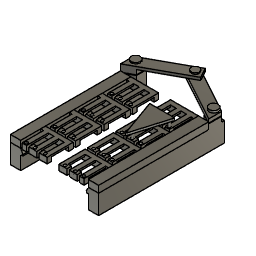
GuitarBuddy (Autodesk Fusion 360 design; units mm, degrees)
Autodesk Fusion 360 part; units mm, degrees
note: some values were not read from the file. Chosen so that the rebuilt part matches the saved one: a direction; which face or edge a step refers to. Set by a fixed rule: which sketch regions a step uses.
sketch "Sketch1" plane through (0, 0, 0) normal (0, 0, 1) x (1, 0, 0)
  line L0 (0, 0) -> (4.5, 0)
  line L1 (4.5, 0) -> (4.5, 101.6)
  line L2 (4.5, 101.6) -> (0, 101.6)
  line L3 (0, 101.6) -> (0, 0)
  line L4 (4.5, 101.6) -> (41, 101.6) construction
  line L5 (41, 101.6) -> (41, 121.6) construction
  line L6 (41, 121.6) -> (4.5, 101.6)
  line L7 (41, 121.6) -> (36.1947, 130.3698)
  line L8 (36.1947, 130.3698) -> (0, 110.5371)
  line L9 (0, 110.5371) -> (0, 101.6)
  line L10 (4.5, 101.6) -> (4.5, 110.5371)
  line L11 (4.5, 110.5371) -> (0, 110.5371)
  line L12 (-4.5, 110.5371) -> (0, 110.5371)
  line L13 (-4.5, 101.6) -> (-4.5, 110.5371)
  line L14 (-4.5, 0) -> (-4.5, 101.6)
  line L15 (0, 0) -> (-4.5, 0)
  line L16 (0, 110.5371) -> (-4.5, 108.0713)
  line L17 (4.5, 101.6) -> (-4.5, 96.6685)
  line L18 (4.5, 101.6) -> (-4.5, 101.6)
  line L19 (34.2124, 123.5822) -> (34.2124, 117.8808) construction
  line L20 (63.9249, 101.6) -> (72.9249, 96.6685)
  line L21 (63.9249, 101.6) -> (72.9249, 101.6) construction
  line L22 (27.4249, 121.6) -> (32.2302, 130.3698)
  line L23 (68.4249, 110.5371) -> (68.4249, 101.6)
  line L24 (63.9249, 110.5371) -> (68.4249, 110.5371)
  line L25 (68.4249, 110.5371) -> (72.9249, 108.0713)
  line L26 (72.9249, 0) -> (72.9249, 101.6)
  line L27 (72.9249, 101.6) -> (72.9249, 110.5371)
  line L28 (63.9249, 101.6) -> (27.4249, 101.6) construction
  line L29 (63.9249, 0) -> (63.9249, 101.6)
  line L30 (68.4249, 101.6) -> (68.4249, 0)
  line L31 (27.4249, 121.6) -> (63.9249, 101.6)
  line L32 (34.2124, 123.5822) -> (34.2124, 117.8808) construction
  line L33 (32.2302, 130.3698) -> (68.4249, 110.5371)
  line L34 (63.9249, 101.6) -> (68.4249, 101.6) construction
  line L35 (72.9249, 110.5371) -> (68.4249, 110.5371)
  line L36 (27.4249, 101.6) -> (27.4249, 121.6) construction
  line L37 (63.9249, 101.6) -> (63.9249, 110.5371)
  line L38 (68.4249, 0) -> (72.9249, 0)
  line L39 (68.4249, 0) -> (63.9249, 0)
  circle A0 centre (34.2124, 123.5822) radius 2.7
  circle A1 centre (34.2124, 123.5822) radius 3
  circle A2 centre (34.2124, 123.5822) radius 3.45
  line L40 (-4.5, 105.5371) -> (4.5, 105.5371) construction
  circle A3 centre (0, 105.5371) radius 3
  circle A4 centre (0, 105.5371) radius 4
  circle A5 centre (0, 105.5371) radius 2.4
  line L41 (72.9249, 105.5371) -> (63.9249, 105.5371) construction
  circle A6 centre (68.4249, 105.5371) radius 2.4
  circle A7 centre (68.4249, 105.5371) radius 3
  circle A8 centre (68.4249, 105.5371) radius 4
  point P0 (68.4249, 0)
  dimension "d3" = 4.5
  dimension "d4" = 101.6
  dimension "d9" = 36.5
  dimension "d11" = 20
  dimension "d13" = 10
  dimension "d19" = 5
  dimension "d20" = 5
  dimension "d300" = 6
  dimension "d301" = 6.9
  dimension "d302" = 5.4
  dimension "d337" = 5
  dimension "d338" = 6
  dimension "d339" = 8
  dimension "d340" = 4.8
  constraint horizontal L0
  constraint vertical L1
  constraint horizontal L2
  constraint vertical L3
  constraint coincident L0.start L3.end
  constraint perpendicular L1 L4
  constraint perpendicular L4 L5
  constraint perpendicular L6 L7
  constraint perpendicular L2 L9
  constraint parallel L6 L8
  constraint perpendicular L4 L10
  constraint perpendicular L9 L11
  constraint symmetric L0.start L9 L3.end
  constraint symmetric L0.end L9 L14.start
  constraint symmetric L1.end L9 L13.start
  constraint symmetric L8.end L9 L11.end
  constraint symmetric L9 L10.end L12.start
  constraint coincident L9 L8.end
  constraint coincident L13 L16.end
  constraint collinear L8 L16
  constraint coincident L14 L17.end
  constraint collinear L6 L17
  constraint coincident L6 L19.end
  constraint vertical L19
  constraint symmetric L0.start L19 L30.end
  constraint symmetric L0.start L19 P0
  constraint symmetric L0.end L19 L29.start
  constraint symmetric L1.end L19 L20.start
  constraint symmetric L2.end L19 L23.end
  constraint symmetric L4.end L19 L28.end
  constraint symmetric L5.end L19 L22.start
  constraint symmetric L7.end L19 L22.end
  constraint symmetric L8.end L19 L23.start
  constraint symmetric L10.end L19 L24.start
  constraint symmetric L12.start L19 L27.end
  constraint symmetric L13.start L19 L21.end
  constraint symmetric L14.start L19 L26.start
  constraint symmetric L16.end L19 L25.end
  constraint symmetric L17.end L19 L20.end
  constraint symmetric L32.start L19 A0.centre
  constraint symmetric L32.end L19 L19.end
  constraint concentric A1 A2
  constraint concentric A0 A2
  constraint coincident L19.start L32.start
  constraint coincident L13 L40.start
  constraint coincident L10 L40.end
  constraint horizontal L40
  constraint midpoint L40 A3.centre
  constraint concentric A3 A4
  constraint concentric A3 A5
  constraint symmetric L19 L40.start L41.start
  constraint symmetric L19 L40.end L41.end
  constraint symmetric L19 A3 A7
  constraint symmetric L19 A4 A8
  constraint symmetric L19 A5 A6
  measures "d3" distance of L0.start L0.end
  measures "d4" distance of L0.start L2.end
  measures "d9" distance of L1.end L4.end
  measures "d11" distance of L4.end L5.end
  measures "d13" distance of L5.end L7.end
  measures "d19" distance of L8 L19.start
  measures "d20" distance of L7 L19.start
  measures "d300" diameter of A1
  measures "d301" diameter of A2
  measures "d302" diameter of A0
  measures "d337" distance of L12 L40
  measures "d338" diameter of A3
  measures "d339" diameter of A4
  measures "d340" diameter of A5
extrude "Extrude2" add sketch "Sketch1" along normal blind 3.175 from surface at 5 contours L3 L14 L17 L18 A4 | L2 L3 L17 L18 A4 | L6 L8 L10 L11 L22 L31 | L2 L9 L10 L11 L18 A4 | L3 L18 A4 | L2 L3 L18 A4 | L2 L9 L18 A3 A4 | L6 L7 L8 L22 L31 L33 | L9 L18 A3 A4 | L9 L13 L16 L18 A4 | L9 A3 A5 | L9 A3 A5 | L7 L8 L33 | L9 A5 | L9 A5 | A2 makes body 1 in component "LeftHandleBar"
extrude "Extrude4" add sketch "Sketch1" along normal mid plane 6.35 from surface at 8.175 separate body contours A0 makes body 2 in component "CenterRivot"
extrude "Extrude5" add sketch "Sketch1" along normal blind 1.5875 from surface at 11.35 separate body contours A0 | A1 | A2 makes body 3 in component "CenterRivot"
extrude "Extrude6" add sketch "Sketch1" against normal blind 1.5875 from surface at 5 separate body contours A0 | A1 | A2 makes body 4 in component "CenterRivot"
extrude "Extrude1" add sketch "Sketch1" against normal blind 17 separate body contours L0 L1 L3 L17 | L2 L3 L17 L18 A4 | L2 L9 L10 L11 L18 A4 | L2 L3 L18 A4 | L2 L9 L18 A3 A4 | L9 A3 A5 | L9 A5 picked at (1.628, 103.2671) picked at (0.5577, 104.777) makes body 5
copy_body "Body->Comp1" bodies 5 removing the originals makes body 6 in component "LeftHandle"
sketch "Sketch2" plane through (4.5, 0, 0) normal (1, 0, 0) x (0, 1, 0)
  line L0 (109.1262, 0) -> (0, 0)
  line L1 (0, 0) -> (0, -19.05)
  line L2 (0, -19.05) -> (109.1262, -19.05)
  line L3 (109.1262, -19.05) -> (109.1262, 0)
  line L4 (0, 0) -> (3.81, 0)
  line L5 (3.81, 0) -> (3.81, -5)
  line L6 (3.81, -5) -> (0, -5)
  line L7 (0, -5) -> (0, 0)
  line L8 (101.6, 0) -> (97.79, 0)
  line L9 (97.79, 0) -> (97.79, -5)
  line L10 (97.79, -5) -> (101.6, -5)
  line L11 (101.6, -5) -> (101.6, 0)
  line L12 (110.5371, 0) -> (0, 0)
  line L13 (0, 0) -> (0, -17)
  line L14 (0, -17) -> (110.5371, -17)
  line L15 (110.5371, -17) -> (110.5371, 0)
  point P0 (101.6, 0)
  dimension "d55" = 3.81
  dimension "d56" = 5
  dimension "d66" = 3.81
  dimension "d67" = 5
  constraint horizontal L4
  constraint vertical L5
  constraint horizontal L6
  constraint vertical L7
  constraint coincident L0.end L1.start
  constraint horizontal L8
  constraint vertical L9
  constraint horizontal L10
  constraint vertical L11
  constraint coincident P0 L8.start
  measures "d55" distance of L0.end L4.end
  measures "d56" distance of L0.end L6.end
  measures "d66" distance of P0 L8.end
  measures "d67" distance of P0 L10.end
extrude "Extrude1'" add sketch "Sketch2" along normal blind 1.905 contours L0 L1 L4 L5 L6 L7 L12 L13 bodies 6 in component "LeftHandle"
extrude "Extrude14" add sketch "Sketch2" along normal blind 2.905 contours L0 L8 L9 L10 L11 L12 bodies 6 in component "LeftHandle"
extrude "Extrude3" add 1 faces at (0, 73.6914, -5.6667) along direction (-1, 0, 0) blind 4.5 separate body on bodies 6 makes body 7 in component "LeftHandle"
chamfer "Chamfer1" distance 3.81 distance2 2.905 1 edges at (7.405, 99.695, 0) measured on face at (7.405, 99.06, -1.6667) on bodies 6 in component "LeftHandle"
chamfer "Chamfer2" distance 3.81 distance2 1.905 1 edges at (6.405, 1.905, 0) measured on face at (6.405, 1.27, -3.3333) on bodies 6 in component "LeftHandle"
ref_plane "WorkPlane1" through (0, 0, -1) normal (0, 0, 1) x (1, 0, 0) in component "LeftHandle"
ref_plane "WorkPlane2" through (0, 0, -4) normal (0, 0, 1) x (1, 0, 0) in component "LeftHandle"
sketch "Sketch6" plane through (0, 0, 0) normal (0, 0, 1) x (1, 0, 0)
  line L0 (4.5, 110.5371) -> (0, 110.5371)
  line L1 (0, 110.5371) -> (0, 0)
  line L2 (0, 0) -> (4.5, 0)
  line L3 (4.5, 3.81) -> (4.5, 97.79)
  line L4 (0, 0) -> (0, 110.5371) construction
  line L5 (0, 110.5371) -> (-4.5, 110.5371)
  line L6 (-4.5, 0) -> (0, 0)
  line L7 (41, 121.6) -> (36.1947, 130.3698)
  line L8 (36.1947, 130.3698) -> (-4.5, 108.0713)
  line L9 (-4.5, 108.0713) -> (-4.5, 96.6685)
  line L10 (-4.5, 96.6685) -> (41, 121.6)
  line L11 (34.2124, 123.5822) -> (34.2124, 96.6685) construction
  line L12 (34.2124, 96.6685) -> (4.5, 96.6685) construction
  line L13 (34.2124, 123.5822) -> (36.2124, 123.5822) construction
  line L14 (36.2124, 123.5822) -> (36.2124, 96.6685) construction
  line L15 (36.2124, 96.6685) -> (34.2124, 96.6685) construction
  line L16 (34.2124, 96.6685) -> (34.2124, 123.5822) construction
  line L17 (34.2124, 123.5822) -> (32.2124, 123.5822) construction
  line L18 (32.2124, 123.5822) -> (32.2124, 96.6685) construction
  line L19 (32.2124, 96.6685) -> (34.2124, 96.6685) construction
  line L20 (34.2124, 96.6685) -> (34.2124, 123.5822) construction
  line L21 (32.2124, 96.6685) -> (36.2124, 96.6685) construction
  line L22 (36.2124, 96.6685) -> (36.2124, 0) construction
  line L23 (36.2124, 0) -> (32.2124, 0) construction
  line L24 (32.2124, 0) -> (32.2124, 96.6685) construction
  line L25 (4.5, 96.6685) -> (32.2124, 96.6685) construction
  line L26 (34.2124, 96.6685) -> (34.2124, 0) construction
  circle A0 centre (34.2124, 123.5822) radius 3
  line L27 (34.2124, 123.5822) -> (34.2124, 117.8808)
  line L28 (4.5, 96.6685) -> (32.2124, 96.6685)
  line L29 (32.2124, 96.6685) -> (32.2124, 92.6685)
  line L30 (32.2124, 92.6685) -> (4.5, 92.6685)
  line L31 (4.5, 92.6685) -> (4.5, 96.6685)
  line L32 (11, 92.6685) -> (7, 92.6685)
  line L33 (7, 92.6685) -> (7, 73.6685)
  line L34 (11, 73.6685) -> (11, 92.6685)
  line L35 (11, 73.6685) -> (7, 73.6685)
  circle A1 centre (9, 75.6685) radius 1.25
  line L36 (-4.5, 96.6685) -> (4.5, 96.6685)
  line L37 (7, 77.6685) -> (11, 77.6685)
  line L38 (9, 77.6685) -> (9, 75.6685) construction
  line L39 (11, 77.6685) -> (11, 73.6685) construction
  line L40 (11, 75.6685) -> (9, 75.6685) construction
  line L41 (20, 73.6685) -> (16, 73.6685)
  line L42 (20, 73.6685) -> (20, 92.6685)
  line L43 (16, 77.6685) -> (20, 77.6685)
  line L44 (16, 92.6685) -> (16, 73.6685)
  circle A2 centre (16.5, 75.6685) radius 1.25
  line L45 (20, 75.6685) -> (16.5, 75.6685) construction
  line L46 (20, 92.6685) -> (16, 92.6685)
  line L47 (20, 77.6685) -> (20, 73.6685) construction
  line L48 (16.5, 77.6685) -> (16.5, 75.6685) construction
  line L49 (29, 73.6685) -> (25, 73.6685)
  line L50 (29, 73.6685) -> (29, 92.6685)
  line L51 (25, 77.6685) -> (29, 77.6685)
  line L52 (25, 92.6685) -> (25, 73.6685)
  circle A3 centre (25.5, 75.6685) radius 1.25
  line L53 (29, 75.6685) -> (25.5, 75.6685) construction
  line L54 (29, 92.6685) -> (25, 92.6685)
  line L55 (29, 77.6685) -> (29, 73.6685) construction
  line L56 (25.5, 77.6685) -> (25.5, 75.6685) construction
  line L57 (-4.5, 96.6685) -> (0, 96.6685)
  line L58 (0, 96.6685) -> (0, 0)
  line L59 (0, 0) -> (-4.5, 0)
  line L60 (-4.5, 0) -> (-4.5, 96.6685)
  line L61 (16, 77.6685) -> (13, 77.6685)
  line L62 (13, 77.6685) -> (13, 73.6685)
  line L63 (13, 73.6685) -> (16, 73.6685)
  line L64 (22, 77.6685) -> (22, 73.6685)
  line L65 (22, 73.6685) -> (25, 73.6685)
  line L66 (25, 77.6685) -> (22, 77.6685)
  line L67 (29, 92.6685) -> (29, 96.6685)
  line L68 (13, 77.6685) -> (20, 77.6685) construction
  line L69 (29, 77.6685) -> (22, 77.6685) construction
  line L70 (4.5, 0) -> (4.5, 3.81)
  line L71 (4.5, 97.79) -> (4.5, 101.6)
  line L72 (4.5, 101.6) -> (4.5, 110.5371)
  dimension "d317" = 2
  dimension "d318" = 2
  dimension "d350" = 4
  dimension "d363" = 4
  dimension "d401" = 2.5
  dimension "d436" = 4
  dimension "d437" = 4
  dimension "d438" = 2.5
  dimension "d439" = 4
  dimension "d440" = 4
  dimension "d441" = 2.5
  dimension "d442" = 4
  dimension "d443" = 5
  dimension "d444" = 5
  dimension "d445" = 2.5
  dimension "d446" = 15
  dimension "d447" = 15
  dimension "d449" = 15
  dimension "d465" = 3
  dimension "d466" = 3
  constraint coincident L3 L12.end
  constraint perpendicular L3 L12
  constraint horizontal L13
  constraint vertical L14
  constraint horizontal L15
  constraint vertical L16
  constraint horizontal L17
  constraint vertical L18
  constraint horizontal L19
  constraint vertical L20
  constraint coincident L12 L18.end
  constraint horizontal L21
  constraint vertical L22
  constraint horizontal L23
  constraint vertical L24
  constraint coincident L14.end L15.start
  constraint midpoint L23 L26.end
  constraint horizontal L28
  constraint vertical L29
  constraint vertical L31
  constraint horizontal L32
  constraint vertical L33
  constraint vertical L34
  constraint horizontal L35
  constraint coincident L9.end L10.start
  constraint horizontal L36
  constraint collinear L24 L29
  constraint coincident L33 L37.start
  constraint coincident L34 L37.end
  constraint perpendicular L34 L37
  constraint midpoint L37 L38.start
  constraint coincident A1.centre L38.end
  constraint perpendicular L37 L38
  constraint midpoint L39 L40.start
  constraint perpendicular L39 L40
  constraint horizontal L46
  constraint vertical L44
  constraint vertical L42
  constraint horizontal L41
  constraint coincident L43.start L44
  constraint coincident L43.end L42
  constraint perpendicular L42 L43
  constraint coincident A2.centre L45.end
  constraint perpendicular L43 L48
  constraint midpoint L45.start L47
  constraint perpendicular L45 L47
  constraint horizontal L54
  constraint vertical L52
  constraint vertical L50
  constraint horizontal L49
  constraint coincident L51.start L52
  constraint coincident L51.end L50
  constraint perpendicular L50 L51
  constraint coincident A3.centre L53.end
  constraint perpendicular L51 L56
  constraint midpoint L53.start L55
  constraint perpendicular L53 L55
  constraint collinear L30 L32
  constraint collinear L30 L46
  constraint collinear L30 L54
  constraint collinear L2 L23
  constraint coincident L11.start L13.start
  constraint horizontal L57
  constraint vertical L58
  constraint horizontal L59
  constraint vertical L60
  constraint coincident L1.end L2.start
  constraint vertical L62
  constraint horizontal L61
  constraint horizontal L63
  constraint coincident L41.end L44.end
  constraint vertical L64
  constraint horizontal L66
  constraint horizontal L65
  constraint coincident L49.end L52.end
  constraint coincident L51.start L66.start
  constraint perpendicular L25 L67
  constraint coincident L12 L67.end
  constraint midpoint L48.start L68
  constraint midpoint L56.start L69
  measures "d317" distance of L11 L14
  measures "d318" distance of L16 L18
  measures "d350" distance of L12.end L30.end
  measures "d363" distance of L32.start L32.end
  measures "d401" diameter of A1
  measures "d436" distance of L35 L37
  measures "d437" distance of L42.end L44.start
  measures "d438" diameter of A2
  measures "d439" distance of L41 L43
  measures "d440" distance of L50.end L52.start
  measures "d441" diameter of A3
  measures "d442" distance of L49 L51
  measures "d443" distance of L34 L44
  measures "d444" distance of L42 L52
  measures "d445" distance of L3 L33
  measures "d446" distance of L30 L37
  measures "d447" distance of L30 L43
  measures "d449" distance of L30 L51
  measures "d465" distance of L62.end L41.end
  measures "d466" distance of L64.end L49.end
extrude "Extrude2'" add sketch "Sketch6" along normal blind 6 separate body contours L1 L2 L3 L31 L36 L58 L70 | L1 L6 L36 L57 L58 L59 L60 makes body 8
copy_body "Body->Comp2" bodies 8 removing the originals makes body 9 in component "FretsPushers"
extrude "Extrude14'" add sketch "Sketch6" against normal blind 5 from surface at 6 separate body contours L3 L28 L30 L31 L32 L46 L54 L67 makes body 10 in component "FretsPushers"
extrude "Extrude4'" add sketch "Sketch6" against normal blind 1.5 from surface at 6 contours L30 L32 L33 L34 L37 | L30 L50 L51 L52 L54 | L33 L34 L35 L37 | L49 L50 L51 L52 A3 | L30 L42 L43 L44 L46 | L52 A3 L64 L65 L66 | L41 L42 L43 L44 A2 | L44 A2 L61 L62 L63 | L52 A3 | L52 A3 | L44 A2 | L44 A2 | A1 bodies 10 in component "FretsPushers"
extrude "Extrude12" add sketch "Sketch6" against normal blind 5 from surface at 6 contours L33 L34 L35 L37 | L49 L50 L51 L52 A3 | L52 A3 L64 L65 L66 | L41 L42 L43 L44 A2 | L44 A2 L61 L62 L63 | L52 A3 | L52 A3 | L44 A2 | L44 A2 | A1 bodies 10 in component "FretsPushers"
extrude "Extrude13" cut sketch "Sketch6" against normal blind 2 from surface at 6 contours L52 A3 | L52 A3 | L44 A2 | L44 A2 | A1 bodies 10 in component "FretsPushers"
pattern_linear "R-Pattern2" count 4 spacing 25 along (0, -1, 0) of "Extrude14'", "Extrude4'", "Extrude12", "Extrude13" makes body 11 at (16.5, 70.3352, 6) makes body 12 at (16.5, 45.3352, 6) makes body 13 at (16.5, 20.3352, 6) in component "FretsPushers"
mirror "MirrorComponent5" about plane through (0, 0, 0) normal (0, 0, 1) of bodies 9 10 11 12 13 makes body 14 at (-1.5, 63.1123, 0) makes body 15 at (16.5, 95.3352, -6) makes body 16 at (16.5, 70.3352, -6) makes body 17 at (16.5, 45.3352, -6) makes body 18 at (16.5, 20.3352, -6) in component "Component17(Mirror)"
mirror "MirrorComponent5'" about plane through (0, 0, 0) normal (0, 0, 1) of bodies 6 7 makes body 19 at (4.5, 69.4424, 13) makes body 20 at (-4.5, 73.6914, 5.6667) in component "LeftHandle(Mirror)"
mirror "MirrorComponent5''" about plane through (0, 0, 0) normal (0, 0, 1) of bodies 1 makes body 21 in component "LeftHandleBar(Mirror)"
extrude "Extrude10" add 1 faces at (12.0187, 111.4417, 8.175) along direction (0, 0, 1) blind 3.175 on bodies 1 bodies 1 in component "LeftHandleBar"
extrude "Extrude14''" cut sketch "Sketch1" along normal blind 4 from surface at 5 contours L6 L8 L10 L11 L22 L31 | L6 L7 L8 L22 L31 L33 | L7 L8 L33 | A2 bodies 1 in component "LeftHandleBar"
extrude "Extrude10'" add sketch "Sketch1" along normal up to surface (11.35 mm away) contours L9 A5 | L9 A5 bodies 6 7 in component "LeftHandle"
extrude "Extrude1''" add sketch "Sketch1" along normal up to surface (8.175 mm away) contours L23 A6 | L23 A6 sketch seen with x (-1, 0, 0) y (0, 1, 0) z (0, 0, -1) at (68.4249, 0, 0) bodies 19 20 in component "LeftHandle(Mirror)"
extrude "Extrude12'" cut sketch "Sketch1" along normal up to surface (11.35 mm away) contours L9 A3 A5 | L9 A3 A5 | L9 A5 | L9 A5 bodies 1 in component "LeftHandleBar"
extrude "Extrude1'''" cut sketch "Sketch1" along normal blind 3.175 from surface at 5 contours L23 A6 A7 | L23 A6 A7 | L23 A6 | L23 A6 sketch seen with x (-1, 0, 0) y (0, 1, 0) z (0, 0, -1) at (68.4249, 0, 0) bodies 21 in component "LeftHandleBar(Mirror)"
extrude "Extrude11" add sketch "Sketch1" along normal blind 1.5875 from surface at 11.35 contours L3 L18 A4 | L2 L3 L18 A4 | L2 L9 L18 A3 A4 | L9 L18 A3 A4 | L9 A3 A5 | L9 A3 A5 | L9 A5 | L9 A5 bodies 6 in component "LeftHandle"
extrude "Extrude2''" add sketch "Sketch1" along normal blind 2.5 from surface at 8.175 contours L23 L30 A7 A8 | L23 L30 A7 A8 | L23 A6 A7 | L23 A6 A7 | L23 A6 | L23 A6 sketch seen with x (-1, 0, 0) y (0, 1, 0) z (0, 0, -1) at (68.4249, 0, 0) bodies 19 in component "LeftHandle(Mirror)"
extrude "Extrude12''" cut 1 faces at (12.9152, 107.2721, 11.35) along direction (0, 0, 1) blind 0.6 on bodies 1 bodies 6 in component "LeftHandle"
extrude "Extrude3'" cut 1 faces at (-3.4518, 105.3383, -8.175) along direction (0, 0, -1) blind 0.6 on bodies 19 bodies 19 in component "LeftHandle(Mirror)"
extrude "Extrude8" cut sketch "Sketch1" against normal blind 0.6 from surface at 5 contours A1 | A2 bodies 4 in component "CenterRivot"
extrude "Extrude9" cut sketch "Sketch1" along normal blind 0.6 from surface at 11.35 contours A1 | A2 bodies 3 in component "CenterRivot"
extrude "Extrude13'" add sketch "Sketch1" along normal blind 4.5 contours L3 L14 L17 L18 A4 | L2 L3 L17 L18 A4 | L2 L9 L10 L11 L18 A4 | L3 L18 A4 | L2 L3 L18 A4 | L2 L9 L18 A3 A4 | L9 L18 A3 A4 | L9 L13 L16 L18 A4 bodies 6 in component "LeftHandle"
extrude "Extrude4''" add sketch "Sketch1" along normal blind 4.5 contours L20 L23 L24 L30 L37 A8 | L20 L23 L25 L26 L27 L30 A8 | L23 L30 A7 A8 | L23 L30 A7 A8 sketch seen with x (-1, 0, 0) y (0, 1, 0) z (0, 0, -1) at (68.4249, 0, 0) bodies 19 in component "LeftHandle(Mirror)"
sketch "Sketch7" plane through (0, 0, 6) normal (0, 0, 1) x (-1, 0, 0)
  line L0 (4.5, 0) -> (-4.5, 0)
  line L1 (-72.9249, 0) -> (-63.9249, 0)
  line L2 (-51.9249, -50.6685) -> (-59.4249, -75.6685)
  line L3 (-59.4249, -75.6685) -> (-42.9249, -75.6685)
  circle A0 centre (-42.9249, -75.6685) radius 0.875
  circle A1 centre (-59.4249, -75.6685) radius 0.875
  circle A2 centre (-51.9249, -50.6685) radius 0.875
  line L4 (-16, -42.6685) -> (-16, -27.6685)
  line L5 (-13, -23.6685) -> (-20, -23.6685)
  line L6 (-20, -23.6685) -> (-20, -42.6685)
  line L7 (-25, -42.6685) -> (-25, -27.6685)
  line L8 (-22, -23.6685) -> (-29, -23.6685)
  line L9 (-29, -23.6685) -> (-29, -46.6685)
  line L10 (4.5, 0) -> (4.5, -96.6685)
  line L11 (4.5, -96.6685) -> (-4.5, -96.6685)
  line L12 (-72.9249, 0) -> (-72.9249, -96.6685)
  line L13 (-72.9249, -96.6685) -> (-63.9249, -96.6685)
  circle A3 centre (-16.5, -25.6685) radius 1.25
  circle A4 centre (-25.5, -25.6685) radius 1.25
  line L14 (-4.5, 0) -> (-4.5, -96.6685)
  line L15 (-63.9249, 0) -> (-63.9249, -96.6685)
  circle A5 centre (-42.9249, -75.6685) radius 1.25
  circle A6 centre (-51.9249, -75.6685) radius 1.25
  circle A7 centre (-59.4249, -75.6685) radius 1.25
  circle A8 centre (-51.9249, -50.6685) radius 1.25
  circle A9 centre (-42.9249, -75.6685) radius 1.25
  circle A10 centre (-51.9249, -75.6685) radius 1.25
  circle A11 centre (-59.4249, -75.6685) radius 1.25
  circle A12 centre (-42.9249, -50.6685) radius 1.25
  circle A13 centre (-51.9249, -50.6685) radius 1.25
  circle A14 centre (-59.4249, -50.6685) radius 1.25
  line L16 (-42.9249, -75.6685) -> (-51.9249, -50.6685)
  line L17 (-40.0792, -77.6685) -> (-52.0976, -44.2841)
  line L18 (-52.0976, -44.2841) -> (-62.113, -77.6685)
  line L19 (-62.113, -77.6685) -> (-40.0792, -77.6685)
  line L20 (-45.7705, -73.6685) -> (-51.7522, -57.0529)
  line L21 (-51.7522, -57.0529) -> (-56.7368, -73.6685)
  line L22 (-56.7368, -73.6685) -> (-45.7705, -73.6685)
  line L23 (-16, -27.6685) -> (-13, -27.6685)
  line L24 (-13, -27.6685) -> (-13, -23.6685)
  line L25 (-25, -27.6685) -> (-22, -27.6685)
  line L26 (-22, -27.6685) -> (-22, -23.6685)
  circle A15 centre (-9, -25.6685) radius 1.25
  line L27 (-29, -46.6685) -> (-4.5, -46.6685)
  line L28 (-4.5, -46.6685) -> (-4.5, -42.6685)
  line L29 (-4.5, -42.6685) -> (-7, -42.6685)
  line L30 (-7, -42.6685) -> (-7, -23.6685)
  line L31 (-7, -23.6685) -> (-11, -23.6685)
  line L32 (-11, -23.6685) -> (-11, -42.6685)
  line L33 (-11, -42.6685) -> (-16, -42.6685)
  line L34 (-20, -42.6685) -> (-25, -42.6685)
  dimension "d429" = 1.75
  dimension "d430" = 1.75
  dimension "d431" = 1.75
  dimension "d463" = 2
  dimension "d464" = -2
  constraint coincident L3.end A0.centre
  constraint coincident L2.end L3.start
  constraint coincident L2.start A2.centre
  measures "d429" diameter of A0
  measures "d430" diameter of A1
  measures "d431" diameter of A2
extrude "Extrude1''''" add sketch "Sketch7" along normal blind 2 from surface at 5 separate body contours L2 A2 L16 | L2 A2 L16 | L2 A2 A8 A13 L16 | L2 A2 A8 A13 L16 | L2 L3 A5 A6 A7 A8 A9 A10 A11 A13 L16 | L2 L3 A1 A7 A11 | L2 L3 A1 A7 A11 | L3 A0 A5 A9 L16 | L3 A0 A5 A9 L16 | L2 L3 A1 | L2 L3 A1 | L3 A0 L16 | L3 A0 L16 | L3 A6 A10 | L3 A6 A10 | L17 L18 L19 | L20 L21 L22 makes body 22 in component "DShapeChord"
extrude "Extrude2'''" add sketch "Sketch7" against normal blind 9 from surface at 7 contours L2 A2 L16 | L2 A2 L16 | L2 L3 A1 | L2 L3 A1 | L3 A0 L16 | L3 A0 L16 bodies 22 in component "DShapeChord"
component "LeftHandleBar" placed x (1, 0, 0) y (0, 1, 0) z (0, 0, 1) at (0, 0, 0)
component "CenterRivot" placed x (1, 0, 0) y (0, 1, 0) z (0, 0, 1) at (0, 0, 0)
component "LeftHandle" placed x (1, 0, 0) y (0, 1, 0) z (0, 0, 1) at (0, 0, 0)
component "FretsPushers" placed x (1, 0, 0) y (0, 1, 0) z (0, 0, 1) at (0, 0, 0)
component "LeftHandleBar(Mirror)" placed x (-1, 0, 0) y (0, 1, 0) z (0, 0, -1) at (68.4249, 0, 0)
component "LeftHandle(Mirror)" placed x (-1, 0, 0) y (0, 1, 0) z (0, 0, -1) at (68.4249, 0, 0)
component "Component17(Mirror)" placed x (-1, 0, 0) y (0, 1, 0) z (0, 0, -1) at (68.4249, 0, 0)
component "DShapeChord" placed x (1, 0, 0) y (0, 1, 0) z (0, 0, 1) at (0, 0, 0)
equation "SideLength = 101.6 mm"
equation "SideThickness = 9 mm"
equation "d3 = SideThickness / 2"
equation "d4 = SideLength"
equation "SideHeight = 17 mm"
equation "FirstFretWidth = 55 mm"
equation "d9 = FirstFretWidth / 2 + SideThickness"
equation "LengthToPivot = 20 mm"
equation "d11 = LengthToPivot"
equation "PivotBarThickness = 10 mm"
equation "d13 = PivotBarThickness"
equation "PivotHoleDiam = 4 mm"
equation "BuddyFretBoardThickness = 6.350 mm"
equation "d17 = BuddyFretBoardThickness / 2"
equation "d19 = PivotHoleInlayDistance"
equation "d20 = PivotHoleInlayDistance"
equation "BasePlaneToNub = 5 mm"
equation "nubLength = 3.810 mm"
equation "d55 = nubLength"
equation "d56 = BasePlaneToNub"
equation "NubThickness = 1.905 mm"
equation "d66 = nubLength"
equation "d67 = BasePlaneToNub"
equation "PivotHoleInlayDistance = 5 mm"
equation "BallJointThinDiam = 2 mm"
equation "BallJointTolerance = 0.6 mm"
equation "BallJointHoldinLayerThickness = 1 mm"
equation "d176 = -SideHeight"
equation "d178 = NubThickness"
equation "d184 = SideThickness / 2"
equation "BallJointBigDiam = 6 mm"
equation "d202 = -BallJointHoldinLayerThickness"
equation "d203 = -3 * BallJointHoldinLayerThickness"
equation "VerticalSpaceBetweenKeys = 4 mm"
equation "HorizontalSpaceBetweenKeys = 4 mm"
equation "StringAboveFretBoardHeight = 2 mm"
equation "d294 = BuddyFretBoardThickness / 4"
equation "d296 = BallJointTolerance"
equation "d300 = BallJointBigDiam"
equation "d301 = BallJointBigDiam * 1.15"
equation "d302 = BallJointBigDiam - BallJointTolerance"
equation "d303 = BuddyFretBoardThickness / 2"
equation "d306 = BuddyFretBoardThickness / 4"
equation "d310 = -BuddyFretBoardThickness / 4"
equation "d316 = PivotBarThickness / 2 - 1 mm"
equation "d317 = BallJointBigDiam / 3"
equation "d318 = BallJointBigDiam / 3"
equation "d324 = PivotBarThickness / 4"
equation "d326 = -BallJointTolerance"
equation "d332 = -BallJointTolerance"
equation "d335 = BallJointTolerance"
equation "d338 = BallJointBigDiam"
equation "d339 = BallJointBigDiam + 2 mm"
equation "d340 = BallJointBigDiam - 2 * BallJointTolerance"
equation "FingerWidth = 4 mm"
equation "FingerStringSpacing = 5 mm"
equation "d350 = FingerWidth"
equation "d363 = FingerWidth"
equation "d367 = -( if(TPUPresser == 1; 2 * 1.5 mm; 1.5 mm) )"
equation "d417 = CenterPivotOffset"
equation "CenterPivotOffset = 5 mm"
equation "d425 = CenterPivotOffset - 0.5 mm"
equation "d436 = FingerWidth"
equation "d437 = FingerWidth"
equation "d439 = FingerWidth"
equation "d440 = FingerWidth"
equation "d442 = FingerWidth"
equation "d443 = FingerStringSpacing"
equation "d444 = FingerStringSpacing"
equation "d445 = FingerStringSpacing / 2"
equation "d446 = FingerLength"
equation "d447 = FingerLength"
equation "FingerLength = 15 mm"
equation "d449 = FingerLength"
equation "d464 = -d463"
equation "TPUPresser = 0" comment "Boolean value for if presser is made of tpu (will increase thickness)"
equation "d468 = NubThickness + 1 mm"
equation "d470 = nubLength"
equation "d471 = NubThickness + 1 mm"
equation "d472 = nubLength"
equation "d474 = CenterPivotOffset - 0.5 mm"
named bodies: "Body67 (2)", "Body67 (4)", "Body67 (6)"
